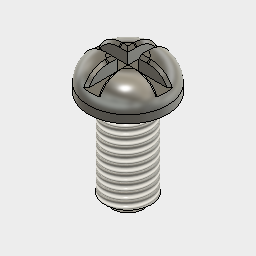
M3x6 Screw (Autodesk Fusion 360 design; units mm, degrees)
Autodesk Fusion 360 part; units mm, degrees
sketch "Sketch1" plane through (0, 0, 0) normal (0, 1, 0) x (1, 0, 0)
  circle A0 centre (0, 0) radius 2.5
  dimension "d1" = 5
  measures "d1" diameter of A0
extrude "Extrude1" add sketch "Sketch1" along normal blind 2
sketch "Sketch2" plane through (0, 0, 0) normal (0, -1, 0) x (1, 0, 0)
  circle A0 centre (0, 0) radius 2.5
  circle A1 centre (0, 0) radius 1.5
  dimension "d4" = 3
  measures "d4" diameter of A1
extrude "Extrude2" add sketch "Sketch2" along normal blind 6 contours A1
fillet "Fillet1" radius 1.5 1 edges at (-2.3308, 2, 0.904)
thread "Thread1" "ISO Metric profile 3.0 M3x0.5 6g" major diameter 2.927 minor diameter 2.3555 pitch 0.5 angle 60 resizes the face on face at (1.4981, -4, -0.0748)
chamfer "Chamfer1" distance 0.5 angle 45 1 edges at (-1.3645, -6, -0.5292)
sketch "Sketch3" plane through (0, 0, 0) normal (1, 0, 0) x (0, 0, -1)
sketch "Sketch4" plane through (0, 2, 0) normal (0, 1, 0) x (-1, 0, 0)
  circle A0 centre (0, 0) radius 1
  line L0 (-2.5, -0.35) -> (2.5, -0.35)
  line L1 (2.5, -0.35) -> (2.5, 0.35)
  line L2 (2.5, 0.35) -> (-2.5, 0.35)
  line L3 (-2.5, 0.35) -> (-2.5, -0.35)
  line L4 (-2.5, -0.35) -> (2.5, 0.35) construction
  line L5 (2.5, -0.35) -> (-2.5, 0.35) construction
  line L6 (-0.35, -2.5) -> (0.35, -2.5)
  line L7 (0.35, -2.5) -> (0.35, 2.5)
  line L8 (0.35, 2.5) -> (-0.35, 2.5)
  line L9 (-0.35, 2.5) -> (-0.35, -2.5)
  line L10 (-0.35, -2.5) -> (0.35, 2.5) construction
  line L11 (0.35, -2.5) -> (-0.35, 2.5) construction
  dimension "d9" = 5
  dimension "d10" = 0.7
  dimension "d11" = 0.7
  dimension "d12" = 5
  measures "d9" distance of L1.end L2.end
  measures "d10" distance of L0.end L1.end
  measures "d11" distance of L7.end L8.end
  measures "d12" distance of L6.end L7.end
extrude "Extrude3" cut sketch "Sketch4" against normal blind 0.883 contours A0 L0 L2 L7 | A0 L0 L1 L2 | A0 L2 L7 L9 | A0 L7 L8 L9 | L0 L2 L7 L9 | A0 L6 L7 L9 | A0 L0 L7 L9 | A0 L0 L2 L9 | A0 L0 L2 L3
chamfer "Chamfer2" distance 0.173 angle 45 14 edges at (-0.35, 1.7659, 1.7673) (-0.35, 2, 0.6434) (-0.6434, 2, 0.35) (-1.7673, 1.7659, 0.35) (-1.7673, 1.7659, -0.35) (-0.6434, 2, -0.35) (-0.35, 2, -0.6434) (-0.35, 1.7659, -1.7673) (0.6434, 2, -0.35) (1.7673, 1.7659, -0.35) (0.35, 2, 0.6434) (0.35, 1.7659, 1.7673) (1.7673, 1.7659, 0.35) (0.6434, 2, 0.35)
